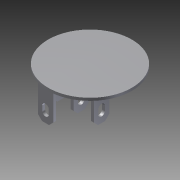
# Autodesk Inventor part: YB16SKW01-05-BBterminal
Saved by Autodesk Inventor 2014 (Build 180170000, 170)
## iProperties
Category: PARTsolutions
Company: NKKSWITCHES
Created: 2013-12-31
Part Number: YB16SKW01-05-BBterminal
Catalog Web Link: www.cadenas.de
Description: Panel Mount Illuminated Pushbuttons_terminal-
Vendor: NKKSWITCHES
Document SubType Name: Modeling
Designer: PARTuser1
Manufacturer: NKKSWITCHES
Density: 1 g/cm^3
Material: Generic
Appearance: RGB(191.25000000000000,191.25000000000000,191.25000000000000)
PSOL_IDENT_0: {$CADENAS_DATA\23d-libs\nkkswitches\pushbuttons\yb\parts\yb_terminal.prj},271 {VTYP=3D},{NB=YB16SKW0
PSOL_IDENT_1: 1-05-BBterminal},{LINA=YB16SKW01-05-BBterminal},{NN=Panel Mount Illuminated Pushbuttons_terminal},{D
PSOL_IDENT_2: ATE=04.07.2008 12:14:55},{GEOMDATE=04.07.2008 00:00:00},{VERSION=},{LINEID=10},{LINESUBID=-1},{WBVAR
PSOL_IDENT_3: =PLS,CRCTS,PS,SHPS,CMR,TRMNLS,LMPS,RSSTR,CTCLR}  {NB=YB16SKW01-05-BBterminal},{LINA=YB16SKW01-05-BBt
PSOL_IDENT_4: erminal},{KT=DUMMY},{PN=YB16SKW01-05-BB},{SRS=YB},{PLS=1},{CRCTS=6},{PS=},{SHPS=S},{SHPSALG= 'S', 'S
PSOL_IDENT_5: - Square (Bushing Mounting)', 'C'  , 'C - Round (Bushing Mounting)', 'R', 'R - Rectangular (Bushing
PSOL_IDENT_6: Mounting)'  , 'K', 'K - Square (Snap-in Mounting)', 'M', 'M - Round (Snap-in Mounting)'  , 'N', 'N
PSOL_IDENT_7: - Rectangular (Snap-in Mounting)' },{HSNG=K - Black only},{CMR=W},{TRMNLS=01},{A=0.709},{A1=0.591},{
PSOL_IDENT_8: A11=0.827},{B=0.709},{B1=0.591},{L=0.669},{L1=0.327},{L2=0.957},{L3=0.429},{L4=0.370},{L5=0.118},{L6
PSOL_IDENT_9: =0.209},{L7=0.157},{DIA1=0.591},{DIA=0.709},{H=0.288},{LMPS=05},{LMPS1= '05','05 - 5-volt (Incandesc
PSOL_IDENT_10: ent Lamp used with Solid Cap)', '12','12 - 12-volt (Incandescent Lamp used with Solid Cap)', '01','0
PSOL_IDENT_11: 1 - 110-volt (Neon used w/ Insert Cap)', '05','05 - 5-volt (Incandescent used w/ Insert Cap)', '12',
PSOL_IDENT_12: '12 - 12-volt (Incandescent used w/ Insert Cap)', '5C','5C - Red (Bright LED used with LED Cap)', '5
PSOL_IDENT_13: D','5D - Amber (Bright LED used with LED Cap)', '5F','5F - Green (Bright LED used with LED Cap)', '6
PSOL_IDENT_14: B','6B - White (Super Bright LED used with LED Cap)', '6F','6F - Green (Super Bright LED used with L
PSOL_IDENT_15: ED Cap)', '6G','6G - Blue (Super Bright LED used with LED Cap)', '1C','1C - Red Single Color (LED in
PSOL_IDENT_16: Spot Illuminated Cap)', '1D','1D - Amber Single Color (LED in Spot Illuminated Cap)', '1F','1F - Gr
PSOL_IDENT_17: een Single Color (LED in Spot Illuminated Cap)', 'CF','CF - Red/Green Bicolor (LED in Spot Illuminat
PSOL_IDENT_18: ed Cap)' },{RSSTR=},{RSSTR1= '','N/A' },{CTCLR=BB},{CTCLR1= 'BB','BB - White/White (Solid Cap: Lens/
PSOL_IDENT_19: Insert Colors)', 'CB','CB - Red/White (Solid Cap: Lens/Insert Colors)', 'EB','EB - Yellow/White (Sol
PSOL_IDENT_20: id Cap: Lens/Insert Colors)', 'FB','FB - Green/White (Solid Cap: Lens/Insert Colors)', 'GB','GB - Bl
PSOL_IDENT_21: ue/White (Solid Cap: Lens/Insert Colors)' },{COL=0.75,0.75,0.75,0.00},{OCHR=Download pdf},{NDM=16.00
PSOL_IDENT_22: 0}
CNS_NN: Panel Mount Illuminated Pushbuttons_terminal
CNS_NB: YB16SKW01-05-BBterminal
CNS_NBSYN: $PN.terminal
CNS_LINA: YB16SKW01-05-BBterminal
CNS_PN: YB16SKW01-05-BB
CNS_SRS: YB
CNS_PLS: 1 - SPDT
CNS_CRCTS: 6 - ON/ON
CNS_PS: Without Panel Seal
CNS_SHPS: S - Square (Bushing Mounting)
CNS_SHPSALG: 'S', 'S - Square (Bushing Mounting)', 'C'  , 'C - Round (Bushing Mounting)', 'R', 'R - Rectangular (Bushing Mounting)'  , 'K', 'K - Square (Snap-in Mounting)', 'M', 'M - Round (Snap-in Mounting)'  , 'N', 'N - Rectangular (Snap-in Mounting)'
CNS_HSNG: K - Black only
CNS_CMR: W - Silver; Rated 3A @ 125V AC
CNS_TRMNLS: 01 - Solder Lug/.110" (2.8mm) Quick Connect
CNS_A: 0.709
CNS_A1: 0.591
CNS_A11: 0.827
CNS_B: 0.709
CNS_B1: 0.591
CNS_L: 0.669
CNS_L1: 0.327
CNS_L2: 0.957
CNS_L3: 0.429
CNS_L4: 0.370
CNS_L5: 0.118
CNS_L6: 0.209
CNS_L7: 0.157
CNS_DIA1: 0.591
CNS_DIA: 0.709
CNS_H: 0.288
CNS_LMPS: 05 - 5-volt (Incandescent Lamp for Solid Cap)
CNS_LMPS1: '05','05 - 5-volt (Incandescent Lamp used with Solid Cap)', '12','12 - 12-volt (Incandescent Lamp used with Solid Cap)', '01','01 - 110-volt (Neon used w/ Insert Cap)', '05','05 - 5-volt (Incandescent used w/ Insert Cap)', '12','12 - 12-volt (Incandescent used w/ Insert Cap)', '5C','5C - Red (Bright LED used with LED Cap)', '5D','5D - Amber (Bright LED used with LED Cap)', '5F','5F - Green (Bright LED used with LED Cap)', '6B','6B - White (Super Bright LED used with LED Cap)', '6F','6F - Green (Super Bright LED used with LED Cap)', '6G','6G - Blue (Super Bright LED used with LED Cap)', '1C','1C - Red Single Color (LED in Spot Illuminated Cap)', '1D','1D - Amber Single Color (LED in Spot Illuminated Cap)', '1F','1F - Green Single Color (LED in Spot Illuminated Cap)', 'CF','CF - Red/Green Bicolor (LED in Spot Illuminated Cap)'
CNS_RSSTR: N/A
CNS_RSSTR1: '','N/A'
CNS_CTCLR: BB - White/White (Solid Cap: Lens/Insert Colors)
CNS_CTCLR1: 'BB','BB - White/White (Solid Cap: Lens/Insert Colors)', 'CB','CB - Red/White (Solid Cap: Lens/Insert Colors)', 'EB','EB - Yellow/White (Solid Cap: Lens/Insert Colors)', 'FB','FB - Green/White (Solid Cap: Lens/Insert Colors)', 'GB','GB - Blue/White (Solid Cap: Lens/Insert Colors)'
CNS_COL: 0.75,0.75,0.75,0.00
CNS_OCHR: Download pdf
CNS_NDM: 16.000
SUPPLIER: NKKSWITCHES
ARTICLENO: YB16SKW01-05-BBterminal
BOMINFO: YB16SKW01-05-BBterminal
CREATOR: CADENAS GmbH
Title: YB16SKW01-05-BBterminal
Author: Cadenas PARTsolutions
Autodesk Inventor part; units mm, degrees
sketch "Sketch_1" plane through (0, 0.508, 0) normal (0, 1, 0) x (1, 0, 0)
  circle A0 centre (0, 0) radius 7.619
  constraints: 1 centre point
extrude "Extrusion1" add sketch "Sketch_1" along normal blind 0.4877
sketch "Sketch_8" plane through (1.8542, 0, 0) normal (1, 0, 0) x (0, 0, -1)
  line L0 (-1.397, -6.5532) -> (-0.635, -7.3152)
  line L1 (-0.635, -7.3152) -> (0.635, -7.3152)
  line L2 (0.635, -7.3152) -> (1.397, -6.5532)
  line L3 (1.397, -6.5532) -> (1.397, 0.762)
  line L4 (1.397, 0.762) -> (-1.397, 0.762)
  line L5 (-1.397, 0.762) -> (-1.397, -6.5532)
  line L6 (-0.5969, -4.8768) -> (-0.5969, -5.6896)
  arc A0 (-0.5969, -5.6896) -> (0.5969, -5.6896) centre (0, -5.6896) ccw
  line L7 (0.5969, -5.6896) -> (0.5969, -4.8768)
  arc A1 (0.5969, -4.8768) -> (-0.5969, -4.8768) centre (0, -4.8768) ccw
  constraints: 16 end point, 4 point on circle, 2 centre point
extrude "Extrusion2" add sketch "Sketch_8" along normal mid plane 0.508
sketch "Sketch_7" plane through (-1.8542, 0, 0) normal (1, 0, 0) x (0, 0, -1)
  line L0 (-1.397, -6.5532) -> (-0.635, -7.3152)
  line L1 (-0.635, -7.3152) -> (0.635, -7.3152)
  line L2 (0.635, -7.3152) -> (1.397, -6.5532)
  line L3 (1.397, -6.5532) -> (1.397, 0.762)
  line L4 (1.397, 0.762) -> (-1.397, 0.762)
  line L5 (-1.397, 0.762) -> (-1.397, -6.5532)
  line L6 (-0.5969, -4.8768) -> (-0.5969, -5.6896)
  arc A0 (-0.5969, -5.6896) -> (0.5969, -5.6896) centre (0, -5.6896) ccw
  line L7 (0.5969, -5.6896) -> (0.5969, -4.8768)
  arc A1 (0.5969, -4.8768) -> (-0.5969, -4.8768) centre (0, -4.8768) ccw
  constraints: 16 end point, 4 point on circle, 2 centre point
extrude "Extrusion3" add sketch "Sketch_7" along normal mid plane 0.508
sketch "Sketch_9" plane through (-5.5499, 0, 0) normal (1, 0, 0) x (0, 0, -1)
  line L0 (-1.397, -6.5532) -> (-0.635, -7.3152)
  line L1 (-0.635, -7.3152) -> (0.635, -7.3152)
  line L2 (0.635, -7.3152) -> (1.397, -6.5532)
  line L3 (1.397, -6.5532) -> (1.397, 0.762)
  line L4 (1.397, 0.762) -> (-1.397, 0.762)
  line L5 (-1.397, 0.762) -> (-1.397, -6.5532)
  line L6 (-0.5969, -4.8768) -> (-0.5969, -5.6896)
  arc A0 (-0.5969, -5.6896) -> (0.5969, -5.6896) centre (0, -5.6896) ccw
  line L7 (0.5969, -5.6896) -> (0.5969, -4.8768)
  arc A1 (0.5969, -4.8768) -> (-0.5969, -4.8768) centre (0, -4.8768) ccw
  constraints: 16 end point, 4 point on circle, 2 centre point
extrude "Extrusion4" add sketch "Sketch_9" along normal mid plane 0.508
sketch "Sketch_2" plane through (0, 0, 4.8514) normal (0, 0, 1) x (1, 0, 0)
  line L0 (-4.3942, -6.5532) -> (-3.6322, -7.3152)
  line L1 (-3.6322, -7.3152) -> (-2.3622, -7.3152)
  line L2 (-2.3622, -7.3152) -> (-1.6002, -6.5532)
  line L3 (-1.6002, -6.5532) -> (-1.6002, 0.762)
  line L4 (-1.6002, 0.762) -> (-4.3942, 0.762)
  line L5 (-4.3942, 0.762) -> (-4.3942, -6.5532)
  line L6 (-3.5941, -4.8768) -> (-3.5941, -5.6896)
  arc A0 (-3.5941, -5.6896) -> (-2.4003, -5.6896) centre (-2.9972, -5.6896) ccw
  line L7 (-2.4003, -5.6896) -> (-2.4003, -4.8768)
  arc A1 (-2.4003, -4.8768) -> (-3.5941, -4.8768) centre (-2.9972, -4.8768) ccw
  constraints: 16 end point, 4 point on circle, 2 centre point
extrude "Extrusion5" add sketch "Sketch_2" along normal mid plane 0.508
sketch "Sketch_11" plane through (0, 0, -4.8514) normal (0, 0, 1) x (1, 0, 0)
  line L0 (-4.3942, -6.5532) -> (-3.6322, -7.3152)
  line L1 (-3.6322, -7.3152) -> (-2.3622, -7.3152)
  line L2 (-2.3622, -7.3152) -> (-1.6002, -6.5532)
  line L3 (-1.6002, -6.5532) -> (-1.6002, 0.762)
  line L4 (-1.6002, 0.762) -> (-4.3942, 0.762)
  line L5 (-4.3942, 0.762) -> (-4.3942, -6.5532)
  line L6 (-3.5941, -4.8768) -> (-3.5941, -5.6896)
  arc A0 (-3.5941, -5.6896) -> (-2.4003, -5.6896) centre (-2.9972, -5.6896) ccw
  line L7 (-2.4003, -5.6896) -> (-2.4003, -4.8768)
  arc A1 (-2.4003, -4.8768) -> (-3.5941, -4.8768) centre (-2.9972, -4.8768) ccw
  constraints: 16 end point, 4 point on circle, 2 centre point
extrude "Extrusion6" add sketch "Sketch_11" along normal mid plane 0.508
ref_plane "terminal_to_body_XY" through (0, 16.9926, 0) normal (0, 1, 0) x (1, 0, 0)
ref_plane "terminal_to_body_YZ" through (0, 16.9926, 0) normal (1, 0, 0) x (0, 0, -1)
ref_plane "terminal_to_body_ZX" through (0, 16.9926, 0) normal (0, 0, -1) x (0, 1, 0)
body "Solid1"
